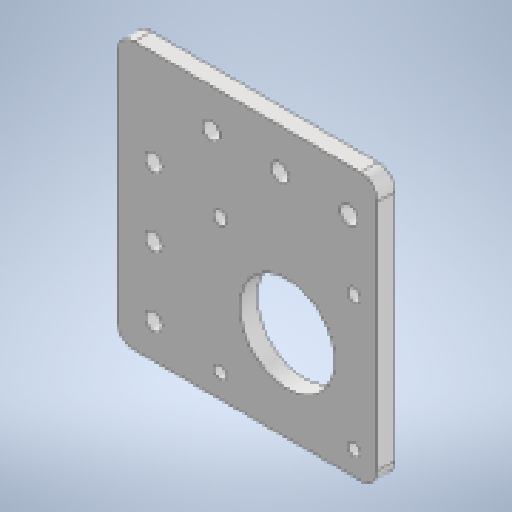
# Autodesk Inventor part: креп_мотора
Saved by Autodesk Inventor 2023.1 (Build 271208000, 208)
## iProperties
Created: 2025-11-24
Part Number: креп_мотора
Material: Типовые
Document SubType Name: Modeling
Designer: DELL
Density: 1 g/cm^3
Appearance: По умолчанию
Author: DELL
Autodesk Inventor part; units mm, degrees
ref_plane "YZ Plane" through (0, 0, 0) normal (1, 0, 0) x (0, 1, 0)
ref_plane "XZ Plane" through (0, 0, 0) normal (0, 1, 0) x (-1, 0, 0)
ref_plane "XY Plane" through (0, 0, 0) normal (0, 0, 1) x (1, 0, 0)
sketch "Эскиз1" plane through (0, 0, 0) normal (0, 0, 1) x (1, 0, 0)
  line L0 (-34.95, 41) -> (-39.5, 41) projected
  line L1 (17, -21) -> (-35.5, -21)
  line L2 (-39.5, -17) -> (-39.5, 37)
  line L3 (-35.5, 41) -> (17, 41)
  line L4 (21, 37) -> (21, -17)
  arc A0 (-39.5, -17) -> (-35.5, -21) centre (-35.5, -17) ccw
  arc A1 (17, -21) -> (21, -17) centre (17, -17) ccw
  arc A2 (21, 37) -> (17, 41) centre (17, 37) ccw
  arc A3 (-35.5, 41) -> (-39.5, 37) centre (-35.5, 37) ccw
  circle A4 centre (-15.5574, -15.5574) radius 1.45 projected
  circle A5 centre (-15.5574, 15.5574) radius 1.45 projected
  circle A6 centre (15.5574, 15.5574) radius 1.45 projected
  circle A7 centre (15.5574, -15.5574) radius 1.45 projected
  line L5 (-34.95, 41) -> (-34.95, -219) construction
  line L6 (-27.05, 41) -> (-27.05, -219) construction
  line L7 (-27.05, -13) -> (-34.95, -13) construction
  circle A8 centre (-31, -13) radius 2
  circle A9 centre (-31, 3) radius 2
  circle A10 centre (-31, 19) radius 2
  line L8 (-35.5, 37) -> (17, -17) construction
  circle A11 centre (14.3534, 31.0936) radius 2
  circle A12 centre (-1.6402, 31.5442) radius 2
  circle A13 centre (-17.6339, 31.9948) radius 2
  point P0 (0, 0)
  point P1 (21, -21)
  dimension "d0" = 4
  dimension "d1" = 8
  dimension "d2" = 4
  dimension "d3" = 4
  dimension "d4" = 4
  dimension "d5" = 16
  dimension "d6" = 16
  constraints: 12 end point, 10 centre point, 8 point on circle, 8 tangent, 6 point on line, 3 equal radius, 3 symmetric about line, 2 horizontal, 2 parallel, 1 midpoint, 1 perpendicular, 3 other
  measures "d0" radius of A0
  measures "d1" distance between parallel lines of L1 L7
  measures "d2" diameter of A8
  measures "d3" diameter of A9
  measures "d4" diameter of A10
  measures "d5" distance of A8.centre A9.centre
  measures "d6" distance of A9.centre A10.centre
extrude "Выдавливание1" add sketch "Эскиз1" along normal blind 4
sketch "Эскиз2" plane through (0, 0, 4) normal (0, 0, 1) x (1, 0, 0)
  circle A0 centre (0, 0) radius 11 projected
  point P0 (0, 0)
extrude "Выдавливание2" cut sketch "Эскиз2" against normal blind 4
